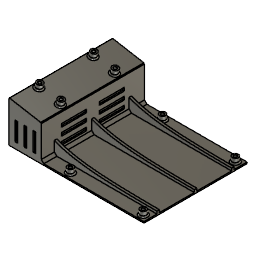
Assembly (Autodesk Fusion 360 archive; units mm, degrees)
design "Chassis"
Autodesk Fusion 360 part; units mm, degrees
sketch "Sketch1" plane through (0, 0, 0) normal (0, 1, 0) x (1, 0, 0)
  line L0 (-52.1948, -64.2034) -> (0, -55)
  line L1 (0, -55) -> (0, 0)
  line L2 (0, 0) -> (165, 0)
  line L3 (165, 0) -> (165, 2.3)
  line L4 (165, 2.3) -> (-52.1948, 2.3)
  line L5 (-52.1948, 2.3) -> (-52.1948, -64.2034)
  dimension "d5" = 165
  dimension "d6" = 2.3
  dimension "d7" = 53
  dimension "d8" = 55
  dimension "d9" = 10
  constraint coincident L1.end L2.start
  constraint vertical L1
  constraint perpendicular L1 L2
  constraint perpendicular L2 L3
  constraint perpendicular L3 L4
  constraint vertical L5
  measures "d5" distance of L1.end L2.end
  measures "d6" distance of L2.end L3.end
  measures "d7" distance of L0.start L0.end
  measures "d8" distance of L0.end L1.end
  measures "d9" angle of L0 L2
extrude "Extrude1" add sketch "Sketch1" along normal mid plane 166
chamfer "Chamfer1" distance 1 angle 45 1 edges at (0, 0, 55)
chamfer "Chamfer3" distance 1 angle 45 1 edges at (-52.1948, 0, 64.2034)
shell "Shell3" thickness 2.3 removed faces 0 bodies 1
sketch "Sketch2" plane through (0, 0, 0) normal (0, 0, 1) x (-1, 0, 0)
  line L0 (0, 83) -> (-165, 83)
  line L1 (-165, 83) -> (-165, -83)
  line L2 (-165, -83) -> (0, -83)
  line L3 (-38, 74) -> (-155, 74) construction
  line L4 (-155, 74) -> (-155, -74) construction
  line L5 (-155, -74) -> (-38, -74) construction
  line L6 (-38, -74) -> (-38, 74) construction
  circle A0 centre (-38, 74) radius 5
  circle A1 centre (-38, -74) radius 5
  circle A2 centre (-155, 74) radius 5
  circle A3 centre (-155, -74) radius 5
  line L7 (0, -83) -> (0, 83)
  point P0 (-38, 0)
  dimension "d14" = 117
  dimension "d15" = 148
  dimension "d17" = 10
  dimension "d18" = 10
  constraint horizontal L3
  constraint vertical L4
  constraint horizontal L5
  constraint vertical L6
  constraint midpoint L6 P0
  constraint horizontal origin P0
  constraint coincident L3.start L6.end
  constraint coincident L5.end L6.start
  constraint equal A0 A1
  constraint coincident L3.end L4.start
  constraint coincident L4.end L5.start
  constraint equal A0 A2
  constraint equal A0 A3
  measures "d14" distance of L3.start L3.end
  measures "d15" distance of L3.start L5.end
  measures "d17" distance of L1 L4
  measures "d18" diameter of A0
extrude "Extrude2" add sketch "Sketch2" along normal blind 8 contours A0 | A1 | A2 | A3
sketch "Sketch3" plane through (9.4056, 0, 53.3415) normal (0.173648, 0, 0.984808) x (0, 1, 0)
  line L0 (83, 10.5506) -> (83, 61.5506)
  line L1 (-83, 61.5506) -> (-83, 10.5506)
  line L2 (-43.5, 53.5506) -> (43.5, 53.5506) construction
  line L3 (43.5, 53.5506) -> (43.5, 18.5506) construction
  line L4 (43.5, 18.5506) -> (-43.5, 18.5506) construction
  line L5 (-43.5, 18.5506) -> (-43.5, 53.5506) construction
  circle A0 centre (-43.5, 53.5506) radius 5
  circle A1 centre (43.5, 53.5506) radius 5
  circle A2 centre (-43.5, 18.5506) radius 5
  circle A3 centre (43.5, 18.5506) radius 5
  line L6 (-83, 10.5506) -> (83, 10.5506)
  line L7 (83, 61.5506) -> (-83, 61.5506)
  point P0 (0, 18.5506)
  point P1 (0, 10.3528)
  dimension "d21" = 87
  dimension "d22" = 35
  dimension "d24" = 10
  dimension "d115" = 8
  constraint horizontal L2
  constraint vertical L3
  constraint horizontal L4
  constraint vertical L5
  constraint midpoint L4 P0
  constraint vertical P0 P1
  constraint coincident L2.start L5.end
  constraint coincident L2.end L3.start
  constraint coincident L4.end L5.start
  constraint coincident L3.end L4.start
  constraint equal A0 A2
  constraint equal A1 A2
  constraint equal A1 A3
  measures "d21" distance of L2.start L2.end
  measures "d22" distance of L2.start L4.end
  measures "d24" diameter of A0
  measures "d115" distance of L2.end L7
extrude "Extrude3" add sketch "Sketch3" along normal blind 8 contours A0 | A1 | A2 | A3
sketch "Sketch5" plane through (10.7947, 0, 61.22) normal (0.173648, 0, 0.984808) x (0, 1, 0)
  circle A0 centre (-43.5, 53.5506) radius 5
  circle A1 centre (43.5, 53.5506) radius 5
  circle A2 centre (-43.5, 18.5506) radius 5
  circle A3 centre (43.5, 18.5506) radius 5
  point P0 (-43.5, 53.5506)
  point P1 (43.5, 53.5506)
  point P2 (43.5, 18.5506)
  point P3 (-43.5, 18.5506)
  constraint coincident P0 A0.centre
  constraint coincident P1 A1.centre
  constraint coincident P2 A3.centre
  constraint coincident A2.centre P3
hole "Hole1" at (-7.4741, -43.5, 64.4413) at (-41.9424, -43.5, 70.519) at (-7.4741, 43.5, 64.4413) at (-41.9424, 43.5, 70.519) direction (-0.173648, 0, -0.984808) diameter 4.5 depth 6 tip angle 180 countersink diameter 5.2 countersink angle 90
sketch "Sketch6" plane through (0, 0, 8) normal (0, 0, 1) x (-1, 0, 0)
  circle A0 centre (-38, 74) radius 5
  circle A1 centre (-38, -74) radius 5
  circle A2 centre (-155, -74) radius 5
  circle A3 centre (-155, 74) radius 5
  point P0 (-38, -74)
  point P1 (-155, -74)
  point P2 (-38, 74)
  point P3 (-155, 74)
  constraint coincident P0 A1.centre
  constraint coincident P1 A2.centre
  constraint coincident P2 A0.centre
  constraint coincident P3 A3.centre
hole "Hole2" at (38, -74, 8) at (38, 74, 8) at (155, 74, 8) at (155, -74, 8) direction (0, 0, -1) diameter 4.5 depth 6 tip angle 180 countersink diameter 5.2 countersink angle 90
fillet "Fillet3" radius 2 4 edges at (42.6616, -75.8081, 0) (42.6616, 72.1919, 0) (159.6616, -75.8081, 0) (159.6616, 72.1919, 0)
fillet "Fillet4" radius 2 4 edges at (-45.1121, 38.8384, 62.9545) (-45.1121, -48.1616, 62.9545) (-10.6439, -48.1616, 56.8768) (-10.6439, 38.8384, 56.8768)
ref_plane "WorkPlane1" through (0, -60, 0) normal (0, 1, 0) x (0, 0, 1)
sketch "Sketch13" plane through (0, -60, 0) normal (0, 1, 0) x (1, 0, 0)
  line L0 (0, 0) -> (0, -54)
  line L1 (165, 0) -> (0, 0)
  spline S0 degree 5 poles (0, -20) (1.8376, -19.2538) (5.6384, -17.8056) (11.7164, -15.7653) (20.5867, -13.3137) (33.034, -10.7197) (46.9512, -8.6162) (62.4322, -6.9976) (79.5092, -5.8106) (98.2078, -4.9827) (118.569, -4.4386) (136.2387, -4.1782) (150.2998, -4.0608) (160.0391, -4.0149) (165, -4) knots 0 0 0 0 0 0 0.1 0.2 0.3 0.4 0.5 0.6 0.7 0.8 0.9 1 1 1 1 1 1
  line L2 (165, -4) -> (165, 0)
  line L3 (142.5764, -4.0673) -> (187.4236, -3.9327)
  point P0 (45.2472, -9.0094)
  dimension "d101" = 4
  dimension "d111" = 20
  constraint coincident L0 S0.start
  constraint coincident L1 L2.end
  constraint perpendicular L1 L2
  constraint midpoint S0.end L3
  constraint coincident L1.start L2.end
  measures "d101" distance of S0.end L1.start
  measures "d111" distance of L0.start S0.start
rib "Rib1" add thickness 4 on both sides direction (-0.096517, 0, -0.995331) up to next extending the curves path "Sketch13" along S0 L2
pattern_linear "R-Pattern4" count 3 spacing 60 along (0, 1, 0) of "Rib1"
chamfer "Chamfer5" distance 4 angle 45 4 edges at (0, -72.5, 0) (0, -30, 0) (0, 30, 0) (0, 72.5, 0)
sketch "Sketch8" plane through (-52.1948, 0, 0) normal (-1, 0, 0) x (0, -1, 0)
  line L0 (-83, 63.2034) -> (-83, -2.3)
  line L1 (-83, -2.3) -> (83, -2.3)
  line L2 (83, -2.3) -> (83, 63.2034)
  line L3 (-50.3935, 12.7) -> (-10.3935, 12.7)
  line L4 (-10.3935, 12.7) -> (-10.3935, 7.7)
  line L5 (-10.3935, 7.7) -> (-50.3935, 7.7)
  line L6 (-50.3935, 7.7) -> (-50.3935, 12.7)
  line L7 (10.3935, 12.7) -> (50.3935, 12.7)
  line L8 (50.3935, 12.7) -> (50.3935, 7.7)
  line L9 (50.3935, 7.7) -> (10.3935, 7.7)
  line L10 (10.3935, 7.7) -> (10.3935, 12.7)
  line L11 (0, 1.75) -> (0, 22.5)
  line L12 (83, 63.2034) -> (-83, 63.2034)
  dimension "d95" = 40
  dimension "d96" = 5
  dimension "d99" = 10
  constraint horizontal L3
  constraint vertical L4
  constraint horizontal L5
  constraint vertical L6
  constraint horizontal L7
  constraint vertical L8
  constraint horizontal L9
  constraint vertical L10
  constraint equal L3 L7
  constraint equal L4 L10
  constraint symmetric L3 L7 L11
  constraint symmetric L4 L10 L11
  measures "d95" distance of L3.start L3.end
  measures "d96" distance of L3.start L5.end
  measures "d99" distance of L1 L5
extrude "Extrude5" cut sketch "Sketch8" against normal blind 90 contours L3 L4 L5 L6 | L7 L8 L9 L10
pattern_linear "R-Pattern1" count 3 spacing 12.5 along (0, 0, 1) of "Extrude5"
sketch "Sketch10" plane through (0, -83, 0) normal (0, -1, 0) x (1, 0, 0)
  line L0 (0, 54) -> (-0.9848, 55.1736)
  line L1 (-0.9848, 55.1736) -> (-51.21, 64.0297)
  line L2 (-52.1948, 63.2034) -> (-52.1948, -2.3)
  line L3 (-52.1948, -2.3) -> (165, -2.3)
  line L4 (165, -2.3) -> (165, 0)
  line L5 (165, 0) -> (4, 0)
  line L6 (0, 4) -> (0, 54)
  line L7 (-42.1948, 37.7) -> (-38.1948, 37.7)
  line L8 (-38.1948, 37.7) -> (-38.1948, 7.7)
  line L9 (-38.1948, 7.7) -> (-42.1948, 7.7)
  line L10 (-42.1948, 7.7) -> (-42.1948, 37.7)
  line L11 (-51.21, 64.0297) -> (-52.1948, 63.2034)
  line L12 (4, 0) -> (0, 4)
  dimension "d76" = 10
  dimension "d78" = 4
  dimension "d94" = 30
  dimension "d113" = 10
  constraint horizontal L7
  constraint vertical L8
  constraint horizontal L9
  constraint vertical L10
  measures "d76" distance of L3 L9
  measures "d78" distance of L7.start L7.end
  measures "d94" distance of L7.end L8.end
  measures "d113" distance of L2 L10
extrude "Extrude7" cut sketch "Sketch10" against normal blind 170 contours L7 L8 L9 L10
pattern_linear "R-Pattern2" count 3 spacing 14.5 along (1, 0, 0) of "Extrude7"
sketch "Sketch9" plane through (0, 0, -2.3) normal (0, 0, -1) x (1, 0, 0)
  line L0 (-52.1948, 83) -> (-52.1948, -83)
  line L1 (-52.1948, -83) -> (165, -83)
  line L2 (165, -83) -> (165, 83)
  line L3 (165, 83) -> (-52.1948, 83)
  circle A0 centre (-26.0974, -30) radius 2.5
  circle A1 centre (-26.0974, 30) radius 2.5
  line L4 (1.75, 0) -> (22.5, 0)
  line L5 (-26.0974, 83) -> (-26.0974, -83) construction
  line L6 (-52.1948, -83) -> (-52.1948, 83)
  line L7 (0, 0) -> (-52.1948, 0) construction
  circle A2 centre (-26.0974, -30) radius 1
  circle A3 centre (-26.0974, 30) radius 1
  dimension "d70" = 5
  dimension "d71" = 60
  dimension "d93" = 2
  constraint equal A0 A1
  constraint symmetric A0 A1 L4
  constraint coincident L3 L5.start
  constraint coincident L1 L5.end
  constraint perpendicular L1 L5
  constraint coincident L7.start origin
  constraint midpoint L6 L7.end
  constraint midpoint L5 L7
  constraint coincident A0.centre L5
  constraint concentric A0 A2
  constraint concentric A1 A3
  constraint equal A2 A3
  measures "d70" diameter of A0
  measures "d71" distance of A0.centre A1.centre
  measures "d93" diameter of A2
extrude "Extrude6" add sketch "Sketch9" along normal up to surface contours A0 | A1 end surface through (-52.1948, 0, 64.2034) normal (0.173648, 0, 0.984808) offset 0
fillet "Fillet5" radius 2 4 edges at (-28.4282, -29.096, 0) (-28.4282, 30.904, 0) (-28.5974, 30, 57.707) (-28.5974, -30, 57.707)

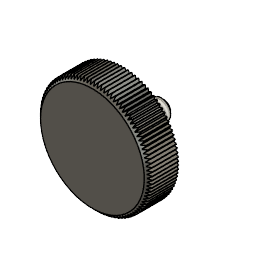
design "Knurled Thumb Screw DIN 653 - M1 x 2 Steel 4.6 Plain"
description: Knurled Thumb Screw DIN 653 - M1 x 2
part number: DIN 653 - M1 x 2 Steel 4.6 Plain
Autodesk Fusion 360 part; units mm, degrees
sketch "Sketch1" plane through (0, 0, 0) normal (0, 1, 0) x (1, 0, 0)
  line L0 (0, 2) -> (0, -1.5)
  line L1 (0, -1.5) -> (-2.55, -1.5)
  line L2 (-2.75, -1.3) -> (-2.75, 0)
  line L3 (-2.75, 0) -> (-1, 0)
  line L4 (-0.5, 0.5) -> (-0.5, 2)
  line L5 (-0.5, 2) -> (0, 2)
  arc A0 (-1, 0) -> (-0.5, 0.5) centre (-1, 0.5) ccw
  line L6 (-2.55, -1.5) -> (-2.75, -1.3)
  dimension "d222" = 1
  dimension "d223" = 2
  dimension "d250" = 0.5
  dimension "d257" = 135
  dimension "d258" = 5.5
  dimension "d259" = 1.5
  dimension "d260" = 0.2
  constraint vertical L0
  constraint coincident L0.end L1
  constraint coincident L0 L1.start
  constraint coincident origin L0
  constraint coincident origin L3
  constraint coincident L0 L5.end
  constraint perpendicular L0 L5
  constraint coincident L0.start L5
  constraint tangent L3 A0
  constraint tangent L4 A0
  constraint horizontal L1
  measures "d223" distance of origin L5
  measures "d250" distance of L4 A0.centre
  measures "d257" angle of L1 L6
  measures "d259" distance of L1 L3
  measures "d260" distance of L1 L2.start
revolve "Revolve1" add sketch "Sketch1" angle 360 about axis through (0, 0, -2) along (0, 0, 1)
sketch "Sketch22" plane through (0, 0, 1.5) normal (0, 0, 1) x (1, 0, 0)
  line L0 (-0.0787, 2.7489) -> (0, 2.6125)
  line L1 (0, 2.6125) -> (0.0787, 2.7489)
  line L2 (0, 0) -> (0, 2.75) construction
  arc A0 (0.0787, 2.7489) -> (-0.0787, 2.7489) centre (0, 0) ccw
  line L3 (0, 0) -> (-2.75, 0) construction
  circle A1 centre (0, 0) radius 2.75
  dimension "d169" = 60
  dimension "d186" = 150
  dimension "d252" = 2.6125
  constraint coincident L0.end L2
  constraint coincident L2.start A0.centre
  constraint coincident A0.centre L2
  constraint vertical L2
  constraint coincident L2.end A0
  constraint coincident L3.end A1
  constraint perpendicular L2 L3
  constraint coincident L2.end A1
  measures "d169" angle of L0 L1
  measures "d186" angle of L0 L2
  measures "d252" distance of L0.end L3
extrude "Extrude11" cut sketch "Sketch22" against normal blind 1.5 contours L0 L1 A0 A1
pattern_circular "C-Pattern4" count 100 over 360 about axis through (0, 0, 1.75) along (0, 0, 1) of "Extrude11"
thread "Thread5" "ISO Metric profile 1.0 M1x0.25 M1x0.25 6g" major diameter 0.9485 minor diameter 0.662 pitch 0.25 angle 60 resizes the face on face at (-0.4975, 0.0498, -1.5)
sketch "Sketch23" plane through (0, 0, 0) normal (0, 1, 0) x (1, 0, 0)
  line L0 (0, 2) -> (0, -1.5)
  line L1 (-0.51, 1.8466) -> (-0.51, 2)
  line L2 (-0.51, 2) -> (0, 2)
  line L3 (-0.51, 1.8466) -> (-0.3466, 2)
  dimension "d254" = 0.51
  dimension "d255" = 0.3466
  dimension "d256" = 0.1534
  constraint coincident L0.start L2.end
  constraint perpendicular L1 L2
  constraint perpendicular L0 L2
  constraint coincident L2 L3.end
  measures "d254" distance of L1 L0.start
  measures "d255" distance of L0 L3.end
  measures "d256" distance of L1.start L2
revolve "Revolve5" cut sketch "Sketch23" angle 360 about axis through (0, 0, 1.75) along (0, 0, 1)
equation "adsk_headdia = 5.50 mm"
equation "adsk_nomdia = 1.00 mm"
equation "adsk_nomlen = 2.00 mm"
equation "adsk_chamheig = 0.20 mm"
equation "d173 = -adsk_headh"
equation "adsk_headh = 1.50 mm"
equation "d222 = adsk_nomdia"
equation "d223 = adsk_nomlen"
equation "adsk_midfillet = 0.50 mm"
equation "adsk_startlen = 0.153363 mm"
equation "adsk_endpointdia = 0.693275 mm"
equation "d250 = adsk_midfillet"
equation "d252 = 0.95 * adsk_headdia / 2"
equation "d254 = adsk_nomdia * 0.51"
equation "d255 = adsk_endpointdia / 2"
equation "d256 = adsk_startlen"
equation "d257 = 180 deg - 45 deg"
equation "d258 = adsk_headdia"
equation "d259 = adsk_headh"
equation "d260 = adsk_chamheig"
